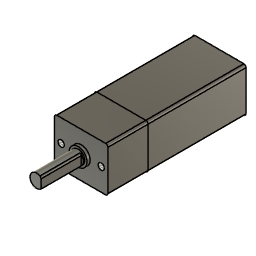
iRob_V1_base v19 (Autodesk Fusion 360 archive; units mm, degrees)
design "N20-Encoder_motor"
Autodesk Fusion 360 part; units mm, degrees
note: some values were not read from the file. Set by a fixed rule: the direction of a hole.
sketch "Sketch1" plane through (0, 0, 0) normal (0, 1, 0) x (1, 0, 0)
  line L0 (0, 0) -> (12, 0)
  line L1 (12, 0) -> (12, -10)
  line L2 (12, -10) -> (0, -10)
  line L3 (0, -10) -> (0, 0)
  circle A0 centre (1.5, -5) radius 0.8
  circle A1 centre (10.5, -5) radius 0.8
  circle A2 centre (6, -5) radius 2
  circle A3 centre (6, -5) radius 1.5
  dimension "d1" = 12
  dimension "d2" = 10
  dimension "d5" = 1.6
  dimension "d6" = 1.6
  dimension "d7" = 4
  dimension "d8" = 3
  constraint horizontal L0
  constraint vertical L1
  constraint horizontal L2
  constraint vertical L3
  constraint coincident L0.start L3.end
  constraint concentric A2 A3
  measures "d1" distance of L0.start L0.end
  measures "d2" distance of L0.start L2.end
  measures "d5" diameter of A0
  measures "d6" diameter of A1
  measures "d7" diameter of A2
  measures "d8" diameter of A3
extrude "Extrude1" add sketch "Sketch1" along normal blind 9 contours L0 L1 L2 L3 | A0 | A1 | A2 | A3 makes body 1
hole "Hole1" at (1.5, 0, 5) direction (0, 1, 0) diameter 1.421 depth 1.2 tip angle 118 bodies 1
thread "Thread1" "ISO Metric profile 1.6 M1.6x0.2 6H" thread offset 0 thread depth 7.4
hole "Hole2" at (10.5, 0, 5) direction (0, 1, 0) diameter 1.421 depth 1.2 tip angle 118 bodies 1
thread "Thread2" "ISO Metric profile 1.6 M1.6x0.2 6H" thread offset 0 thread depth 7.4
extrude "Extrude2" add sketch "Sketch1" against normal blind 0.7 contours A2 bodies 1
extrude "Extrude3" add sketch "Sketch1" against normal blind 10 contours A3 bodies 1
sketch "Sketch2" plane through (0, -10, 0) normal (0, -1, 0) x (1, 0, 0)
  circle A0 centre (6, 5) radius 1.5
  line L0 (4.5, 4.9884) -> (7, 5.0005)
  line L1 (7, 5.0005) -> (5.75, 4.9944)
  line L2 (7, 5.0005) -> (6.9946, 6.1229)
  line L3 (7, 5.0005) -> (7.0054, 3.8868)
  dimension "d25" = 2.5
  constraint coincident A0 L0.start
  constraint parallel L0 L1
  constraint coincident A0 L2.end
  constraint perpendicular L0 L2
  constraint coincident A0 L3.end
  constraint perpendicular L1 L3
  measures "d25" distance of L0.start L0.end
extrude "Extrude4" cut sketch "Sketch2" against normal blind 9 contours A0 L2 L3 bodies 1
fillet "Fillet1" radius 0.5 2 edges at (6.9946, -5.5, 6.1229) (0, 4.5, 10) on bodies 1
fillet "Fillet2" radius 0.5 1 edges at (12, 4.5, 10) on bodies 1
fillet "Fillet3" radius 0.5 1 edges at (12, 4.5, 0) on bodies 1
fillet "Fillet4" radius 0.5 1 edges at (0, 4.5, 0) on bodies 1
extrude "Extrude5" add 1 faces at (4.1667, 9, 6.6667) along direction (0, 1, 0) blind 22 separate body on bodies 1 makes body 2
named bodies: "Gearbox", "DCmotor"

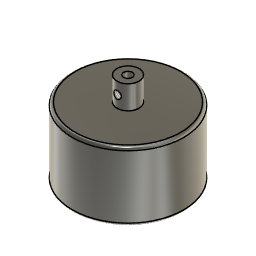
design "38mm Omni Simplified"
Autodesk Fusion 360 part; units mm, degrees
sketch "Sketch1" plane through (0, 0, 0) normal (0, 0, 1) x (1, 0, 0)
  circle A0 centre (0, 0) radius 19
  dimension "d1" = 38
  constraint coincident A0.centre origin
  measures "d1" diameter of A0
extrude "Extrude1" add sketch "Sketch1" along normal blind 24.3
sketch "Sketch2" plane through (0, 0, 24.3) normal (0, 0, 1) x (-1, 0, 0)
  circle A0 centre (0, 0) radius 19
  circle A1 centre (0, 0) radius 4.6188
  dimension "d4" = 9.2376
  constraint coincident A0.centre A1.centre
  measures "d4" diameter of A1
extrude "Extrude2" add sketch "Sketch2" along normal blind 9 contours A1
sketch "Sketch3" plane through (0, 0, 33.3) normal (0, 0, 1) x (-1, 0, 0)
  circle A0 centre (0, 0) radius 4.6188
  circle A1 centre (0, 0) radius 1.5
  dimension "d7" = 3
  constraint coincident A0.centre A1.centre
  measures "d7" diameter of A1
extrude "Extrude3" cut sketch "Sketch3" against normal blind 10 contours A1
move_face "OffsetFaces1" offset -0.869 1 faces at (-4.6131, 0.2302, 30.3)
move_face "OffsetFaces2" offset -1 1 faces at (-2.9859, -0.1863, 33.3)
hole "Hole1" at (0, -3.7498, 28.3) direction (0, 1, 0) diameter 2.529 depth 3 tip angle 118
thread "Thread1" "ISO Metric profile 3.0 M3x0.5 6H" thread offset 0 thread depth 7.4
move_face "OffsetFaces3" offset -0.9 1 faces at (0.3481, 5.4848, 0)
fillet "Fillet1" radius 1 1 edges at (-17.7142, -6.8707, 24.3)
fillet "Fillet2" radius 1 1 edges at (-17.7142, -6.8707, 0.9)
